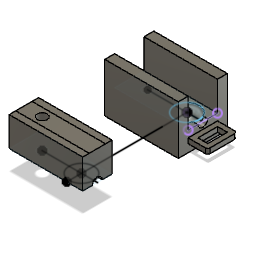
bowden_cable_motor_attachment (Autodesk Fusion 360 design; units mm, degrees)
Autodesk Fusion 360 part; units mm, degrees
note: some values were not read from the file. Set by a fixed rule: which sketch regions a step uses.
sketch "Sketch1" plane through (0, 0, 0) normal (1, 0, 0) x (0, 0, -1)
  line L0 (0, 0) -> (10, 0)
  line L1 (10, 0) -> (10, -10)
  line L2 (10, -10) -> (0, -10)
  line L3 (0, -10) -> (0, 0)
  line L4 (0, 0) -> (10, -10)
  line L5 (0, -10) -> (10, 0)
  line L6 (5, -5) -> (5, 0)
  line L7 (5, 0) -> (10, -10)
  line L8 (6.6667, -3.3333) -> (6.6667, 0)
  line L9 (6.6667, -10) -> (6.6667, -3.3333)
  line L10 (10, 0) -> (6.6667, -10)
  line L11 (8, -6) -> (6.6667, 0)
  line L12 (8, -6) -> (5, -6)
  line L13 (2, -6) -> (3.3333, 0)
  line L14 (2, -6) -> (5, -6)
  dimension "d1" = 10
  dimension "d2" = 10
  constraint horizontal L0
  constraint vertical L1
  constraint horizontal L2
  constraint vertical L3
  constraint coincident L0.start L3.end
  constraint midpoint L4 L6.start
  constraint midpoint L0 L6.end
  constraint coincident L5 L8.start
  constraint coincident L7 L8.start
  constraint coincident L0 L8.end
  constraint perpendicular L0 L8
  constraint coincident L2 L9.start
  constraint perpendicular L2 L9
  constraint coincident L7 L11.start
  constraint coincident L10 L11.start
  constraint horizontal L12
  constraint symmetric L6 L8.end L13.end
  constraint symmetric L6 L11.start L13.start
  constraint symmetric L6 L12.end L14.end
  measures "d1" distance of L0.start L0.end
  measures "d2" distance of L0.start L2.end
extrude "Extrude1" add sketch "Sketch1" along normal blind 15 contours L3 L4 L5 L13 L14 | L0 L4 L13 | L2 L4 L5 L9 L12 L14 | L2 L4 L10 | L4 L9 L10 | L0 L5 L11 | L1 L7 L10 | L4 L7 L10 | L4 L9 L10 L12 | L4 L9 L12 | L5 L10 L11 makes body 1
sketch "Sketch2" plane through (0, -6, 0) normal (0, 1, 0) x (-1, 0, 0)
  line L0 (0, -8) -> (0, -2)
  line L1 (0, -2) -> (-15, -2)
  line L2 (-15, -2) -> (-15, -8)
  line L3 (-15, -8) -> (0, -8)
  line L4 (-15, -2) -> (0, -2)
  line L5 (0, -2) -> (0, -8)
  line L6 (0, -8) -> (-15, -8)
  line L7 (-15, -8) -> (-15, -2)
  line L8 (-15, -2) -> (0, -8)
  line L9 (-15, -8) -> (0, -2)
  line L10 (-7.5, -5) -> (0, -5)
  circle A0 centre (-3.75, -5) radius 1
  dimension "d5" = 2
  constraint horizontal L4
  constraint vertical L5
  constraint horizontal L6
  constraint vertical L7
  constraint coincident L0.start L3.end
  constraint coincident L1.end L2.start
  constraint coincident L2.end L3.start
  constraint coincident L0.end L1.start
  constraint midpoint L9 L10.start
  constraint midpoint L5 L10.end
  constraint midpoint L10 A0.centre
  measures "d5" diameter of A0
extrude "Extrude2" cut sketch "Sketch2" against normal blind 10 contours L10 A0 | L10 A0 bodies 1
sketch "Sketch3" plane through (0, -6, 0) normal (0, 1, 0) x (-1, 0, 0)
  circle A0 centre (-3.75, -5) radius 1
  line L0 (0, -8) -> (0, -2)
  line L1 (0, -2) -> (-15, -2)
  line L2 (-15, -2) -> (-15, -8)
  line L3 (-15, -8) -> (0, -8)
  line L4 (-3.75, -5) -> (-15, -5)
  circle A1 centre (-11.7612, -5) radius 2.5
  dimension "d8" = 5
  constraint coincident A0.centre L4.start
  constraint midpoint L2 L4.end
  constraint coincident L4 A1.centre
  measures "d8" diameter of A1
sphere "SpherePrimitive1" cut diameter 5 placed x (-1, 0, 0) y (0, 0, 1) z (0, 1, 0) at (11.7612, -6, -5) bodies 1
sketch "Sketch4" plane through (0, 0, 0) normal (1, 0, 0) x (0, 0, -1)
  line L0 (0, 0) -> (-11.5117, 0)
  line L1 (-11.5117, 0) -> (-21.5117, 0)
  line L2 (-21.5117, 0) -> (-21.5117, -10)
  line L3 (-21.5117, -10) -> (-11.5117, -10)
  line L4 (-11.5117, -10) -> (-11.5117, 0)
  line L5 (-16.5117, -5) -> (-16.5117, 0)
  line L6 (-18.1783, -3.3333) -> (-18.1783, 0)
  line L7 (4.9359, -6.009) -> (-27.7076, -6.009)
  line L8 (-16.5117, -5) -> (-21.5117, -5)
  line L9 (10, -10) -> (0, -10)
  line L10 (7.5, -6) -> (2.5, -6)
  line L11 (-19.0117, -10) -> (-19.0117, -6)
  line L12 (-21.5117, 0) -> (-18.1783, 0)
  line L13 (-21.5117, -5.9998) -> (-19.5117, -5.9998)
  line L14 (-19.5117, -5.9998) -> (-18.1783, 0)
  line L15 (-13.5117, -5.9998) -> (-14.845, 0)
  line L16 (-37.9592, -6.009) -> (-5.3157, -6.009)
  line L17 (-13.5117, -5.9998) -> (-19.5117, -5.9998)
  line L18 (-13.5117, -5.9998) -> (-19.5117, -5.9998)
  dimension "d10" = 10
  dimension "d11" = 10
  dimension "d12" = 4
  dimension "d13" = 4
  dimension "d14" = 2
  constraint coincident L0.start origin
  constraint horizontal L0
  constraint horizontal L1
  constraint vertical L2
  constraint horizontal L3
  constraint vertical L4
  constraint midpoint L1 L5.end
  constraint coincident L3 L11.start
  constraint coincident L1 L6.end
  constraint perpendicular L1 L6
  constraint horizontal L7
  constraint midpoint L2 L8.end
  constraint perpendicular L7 L11
  constraint coincident L2 L13.start
  constraint perpendicular L2 L13
  constraint symmetric L5 L6.end L15.end
  constraint symmetric L5 L7.start L16.start
  constraint symmetric L5 L7.end L16.end
  constraint symmetric L5 L13.end L15.start
  measures "d10" distance of L0.end L1.end
  measures "d11" distance of L0.end L3.end
  measures "d12" distance of L9 L10
  measures "d13" distance of L11.start L11.end
  measures "d14" distance of L13.start L13.end
extrude "Extrude3" add sketch "Sketch4" along normal blind 15 separate body contours L1 L5 L8 L14 L15 L17 L18 | L1 L5 L8 L14 makes body 2
sketch "Sketch5" plane through (0, -5.9998, 0) normal (0, -1, 0) x (1, 0, 0)
  line L0 (0, 19.5117) -> (0, 13.5117)
  line L1 (0, 13.5117) -> (15, 13.5117)
  line L2 (15, 13.5117) -> (15, 19.5117)
  line L3 (15, 19.5117) -> (0, 19.5117)
  line L4 (0, 19.5117) -> (15, 13.5117)
  line L5 (0, 16.5117) -> (15, 16.5117)
  line L6 (0, -8) -> (0, -2)
  line L7 (0, 16.5117) -> (3.75, 16.5117)
  circle A0 centre (3.75, 16.5117) radius 1
  line L8 (11.7612, -5) -> (11.7612, 16.5117)
  point P0 (3.75, -5)
  point P1 (11.7612, -5)
  point P2 (15, -5)
  dimension "d17" = 3.75
  dimension "d18" = 3.2388
  dimension "d19" = 3.75
  dimension "d20" = 2
  constraint coincident L0.start L3.end
  constraint coincident L1.end L2.start
  constraint midpoint L0 L5.start
  constraint midpoint L2 L5.end
  constraint perpendicular L0 L7
  constraint coincident L7.end A0.centre
  constraint coincident P1 L8.start
  constraint coincident L5 L8.end
  constraint perpendicular L5 L8
  measures "d17" distance of P0 L6
  measures "d18" distance of P1 P2
  measures "d19" distance of L5.start L7.end
  measures "d20" diameter of A0
extrude "Extrude4" cut sketch "Sketch5" against normal blind 15 contours L5 L7 A0 | L5 L7 A0 bodies 2
sketch "Sketch6" plane through (0, -5.9998, 0) normal (0, -1, 0) x (1, 0, 0)
  circle A0 centre (3.75, 16.5117) radius 1
  line L0 (0, 19.5117) -> (0, 13.5117)
  line L1 (0, 13.5117) -> (15, 13.5117)
  line L2 (15, 13.5117) -> (15, 19.5117)
  line L3 (15, 19.5117) -> (0, 19.5117)
  line L4 (15, -2) -> (15, -8)
  line L5 (11.7612, -5) -> (11.7612, 19.5117)
  line L6 (3.75, 16.5117) -> (15, 16.5117)
  circle A1 centre (11.7612, 16.5117) radius 2.5
  point P0 (11.7612, -5)
  dimension "d23" = 3.2388
  dimension "d24" = 5
  constraint coincident P0 L5.start
  constraint coincident L3 L5.end
  constraint perpendicular L3 L5
  constraint coincident A0.centre L6.start
  constraint midpoint L2 L6.end
  constraint coincident L5 A1.centre
  constraint coincident L6 A1.centre
  measures "d23" distance of P0 L4
  measures "d24" diameter of A1
sphere "SpherePrimitive2" cut diameter 5 placed x (1, 0, 0) y (0, 0, 1) z (0, -1, 0) at (11.7612, -5.9998, 16.5117) bodies 2
sketch "Sketch7" plane through (15, 0, 0) normal (1, 0, 0) x (0, 0, -1)
  line L0 (8, -6) -> (2, -6)
  line L1 (2, -6) -> (3.3333, 0)
  line L2 (3.3333, 0) -> (0, 0)
  line L3 (0, 0) -> (0, -10)
  line L4 (0, -10) -> (10, -10)
  line L5 (10, -10) -> (10, 0)
  line L6 (10, 0) -> (6.6667, 0)
  line L7 (6.6667, 0) -> (8, -6)
  circle A0 centre (5, -6) radius 1
  dimension "d26" = 2
  constraint midpoint L0 A0.centre
  measures "d26" diameter of A0
extrude "Extrude5" cut sketch "Sketch7" against normal blind 1 contours L0 A0 picked at (5.3333, -6.4534) bodies 1
sketch "Sketch8" plane through (15, 0, 0) normal (1, 0, 0) x (0, 0, -1)
  arc A0 (4, -6) -> (6, -6) centre (5, -6) ccw
  line L0 (4, -6) -> (2, -6)
  line L1 (2, -6) -> (3.3333, 0)
  line L2 (3.3333, 0) -> (0, 0)
  line L3 (0, 0) -> (0, -10)
  line L4 (0, -10) -> (10, -10)
  line L5 (10, -10) -> (10, 0)
  line L6 (10, 0) -> (6.6667, 0)
  line L7 (6.6667, 0) -> (8, -6)
  line L8 (8, -6) -> (6, -6)
  line L9 (2, -6) -> (2, 0)
  line L10 (8, -6) -> (8, 0)
  line L11 (2, 0) -> (3.3333, 0)
  line L12 (2, -6) -> (3.3333, 0)
  line L13 (6.6667, 0) -> (8, -6)
  line L14 (6.6667, 0) -> (8, 0)
  constraint coincident L0.end L1.start
  constraint coincident L2 L9.end
  constraint perpendicular L2 L9
  constraint coincident L7.end L8.start
  constraint coincident L6 L10.end
  constraint perpendicular L6 L10
  constraint coincident L1.end L2.start
  constraint coincident L6.end L7.start
extrude "Extrude6" cut sketch "Sketch8" against normal blind 15 contours L1 L2 L9 L11 L12 | L6 L7 L10 L13 L14 bodies 1
sketch "Sketch9" plane through (15, 0, 0) normal (1, 0, 0) x (0, 0, -1)
  line L0 (-14.845, 0) -> (-18.1783, 0)
  line L1 (-18.1783, 0) -> (-19.5117, -5.9998)
  line L2 (-19.5117, -5.9998) -> (-13.5117, -5.9998)
  line L3 (-13.5117, -5.9998) -> (-14.845, 0)
  line L4 (-13.5117, -5.9998) -> (-13.5117, 0.0002)
  line L5 (-19.5117, -5.9998) -> (-19.5117, 0.0002)
  line L6 (-19.5117, 0.0002) -> (-18.1783, 0)
  line L7 (-19.5117, -5.9998) -> (-18.1783, 0)
  line L8 (-13.5117, 0.0002) -> (-14.845, 0)
  line L9 (-14.845, 0) -> (-13.5117, -5.9998)
  dimension "d31" = 6
  dimension "d32" = 6
  constraint coincident L2.end L3.start
  constraint perpendicular L2 L4
  constraint coincident L1.end L2.start
  constraint perpendicular L2 L5
  constraint coincident L0.end L1.start
  constraint coincident L0.start L3.end
  measures "d31" distance of L2.end L4.end
  measures "d32" distance of L1.end L5.end
extrude "Extrude7" add sketch "Sketch9" against normal blind 15 contours L3 L4 L8 L9 | L1 L5 L6 L7 bodies 2
sketch "Sketch10" plane through (15, 0, 0) normal (1, 0, 0) x (0, 0, -1)
  line L0 (-14.845, 0) -> (-18.1783, 0)
  line L1 (-18.1783, 0) -> (-19.5117, 0.0002)
  line L2 (-19.5117, 0.0002) -> (-19.5117, -5.9998)
  line L3 (-19.5117, -5.9998) -> (-13.5117, -5.9998)
  line L4 (-13.5117, -5.9998) -> (-13.5117, 0.0002)
  line L5 (-13.5117, 0.0002) -> (-14.845, 0)
  circle A0 centre (-16.5117, -5.9998) radius 1
  dimension "d35" = 2
  constraint midpoint L3 A0.centre
  measures "d35" diameter of A0
extrude "Extrude8" cut sketch "Sketch10" against normal blind 1 contours L3 A0 picked at (-16.4375, -5.6748) bodies 2
sketch "Sketch11" plane through (15, 0, 0) normal (1, 0, 0) x (0, 0, -1)
  line L0 (2, -6) -> (2, 0)
  line L1 (2, 0) -> (0, 0)
  line L2 (0, 0) -> (0, -10)
  line L3 (0, -10) -> (10, -10)
  line L4 (10, -10) -> (10, 0)
  line L5 (10, 0) -> (8, 0)
  line L6 (8, 0) -> (8, -6)
  line L7 (8, -6) -> (6, -6)
  arc A0 (4, -6) -> (6, -6) centre (5, -6) ccw
  line L8 (4, -6) -> (2, -6)
  line L9 (4, -6) -> (4, -10)
  line L10 (5, -7) -> (5, -7.2252)
  line L11 (5, -7.2252) -> (5, -10)
  line L12 (2, -6) -> (2, -10)
  line L13 (8, -6) -> (8, -10)
  line L14 (2, -7.3711) -> (8, -7.3711)
  line L15 (2, -8.393) -> (8, -8.393)
  constraint coincident A0.start L8.start
  constraint coincident L3 L9.end
  constraint tangent A0 L9
  constraint midpoint A0 L10.start
  constraint perpendicular L3 L10
  constraint midpoint L3 L11.end
  constraint perpendicular L3 L11
  constraint coincident L0.start L8.end
  constraint coincident L3 L12.end
  constraint perpendicular L3 L12
  constraint coincident L6.end L7.start
  constraint coincident L3 L13.end
  constraint perpendicular L3 L13
  constraint coincident L12 L14.start
  constraint coincident L13 L14.end
  constraint perpendicular L13 L14
  constraint coincident L12 L15.start
  constraint coincident L13 L15.end
  constraint perpendicular L13 L15
extrude "Extrude9" add sketch "Sketch11" along normal blind 4 contours L9 L12 L14 L15 | L9 L11 L14 L15 | L11 L13 L14 L15 bodies 1
sketch "Sketch12" plane through (0, -7.3711, 0) normal (0, 1, 0) x (-1, 0, 0)
  line L0 (-15, -8) -> (-15, -2)
  line L1 (-15, -2) -> (-19, -2)
  line L2 (-19, -2) -> (-19, -8)
  line L3 (-19, -8) -> (-15, -8)
  line L4 (-16, -3) -> (-18, -3)
  line L5 (-18, -3) -> (-18, -7)
  line L6 (-18, -7) -> (-16, -7)
  line L7 (-16, -7) -> (-16, -3)
  dimension "d40" = -1
extrude "Extrude10" cut sketch "Sketch12" against normal blind 2 contours L4 L5 L6 L7 bodies 1
fillet "Fillet1" radius 0.5 1 edges at (19, -7.882, -8) on bodies 1
fillet "Fillet2" radius 0.5 1 edges at (19, -7.882, -2) on bodies 1
